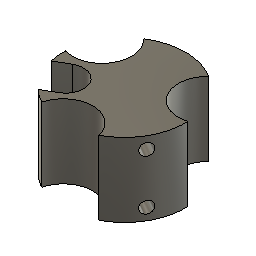
Holder UV v2 (Autodesk Fusion 360 design; units mm, degrees)
Autodesk Fusion 360 part; units mm, degrees
sketch "Sketch1" plane through (0, 0, 0) normal (0, 1, 0) x (1, 0, 0) in component "Holder UV"
  circle A0 centre (0, 0) radius 20.75
  line L0 (0, 0) -> (0, 20.75) construction
  line L1 (0, 0) -> (17.97, -10.375) construction
  line L2 (0, 0) -> (-17.97, -10.375) construction
  circle A1 centre (-12.6656, -7.3125) radius 6.125
  line L3 (-12.6656, -7.3125) -> (-15.7281, -2.0081)
  line L4 (-15.7281, -2.0081) -> (-20.2318, -4.6083)
  line L5 (-12.6656, -7.3125) -> (-9.6031, -12.6169)
  line L6 (-9.6031, -12.6169) -> (-14.1068, -15.2171)
  line L7 (17.97, 10.375) -> (0, -20.75)
  line L8 (0, -20.75) -> (-17.97, 10.375)
  line L9 (17.97, 10.375) -> (-17.97, 10.375)
  circle A2 centre (17.97, 10.375) radius 10
  circle A3 centre (-17.97, 10.375) radius 10
  circle A4 centre (0, -20.75) radius 10
  dimension "d1" = 41.5
  dimension "d4" = 120
  dimension "d5" = 120
  dimension "d6" = 12.25
  dimension "d7" = 6.125
  dimension "d8" = 20
  dimension "d10" = 360
  constraint coincident A0.centre L0.start
  constraint coincident A0 L0.end
  constraint vertical L0
  constraint coincident A0 L1.end
  constraint coincident A0 L2.end
  constraint coincident L2 A1.centre
  constraint coincident A1.centre L3.start
  constraint coincident A1 L3.end
  constraint perpendicular L2 L3
  constraint coincident A0 L4.end
  constraint tangent A1 L4
  constraint symmetric L2 A1.centre L3.start
  constraint symmetric L2 L3.end L5.end
  constraint symmetric L2 L4.end L6.end
  constraint coincident A0 L7.start
  constraint coincident A0 L7.end
  constraint perpendicular L1 L7
  constraint coincident A0 L8.end
  constraint perpendicular L2 L8
  constraint horizontal L9
  constraint coincident L7.start L9.start
  measures "d1" diameter of A0
  measures "d4" angle of L0 L1
  measures "d5" angle of L0 L2
  measures "d6" diameter of A1
  measures "d7" distance of L2.end A1.centre
  measures "d8" diameter of A2
extrude "Extrude1" add sketch "Sketch1" along normal blind 25 contours A0 L7 A2 A4 | A1 L7 L8 L9 A2 A3 A4 | A0 L9 A2 A3 | A0 A1 L6 L8 A4 | A0 A1 L4 L8 A3 in component "Holder UV"
ref_plane "WorkPlane1" through (17.97, 0, 10.375) normal (0.866025, 0, 0.5) x (0, 1, 0) in component "Holder UV"
sketch "Sketch2" plane through (17.97, 0, 10.375) normal (0.866025, 0, 0.5) x (0, 1, 0) in component "Holder UV"
  line L0 (0, -11.0305) -> (0, 11.0305)
  line L1 (0, -11.0305) -> (25, -11.0305)
  line L2 (25, -11.0305) -> (25, 11.0305)
  line L3 (25, 11.0305) -> (0, 11.0305)
  line L4 (0, 0) -> (25, 0) construction
  circle A0 centre (21, 0) radius 2
  circle A1 centre (4, 0) radius 2
  dimension "d11" = 4
  dimension "d12" = 4
  dimension "d13" = 4
  dimension "d14" = 4
  constraint coincident L4.start origin
  constraint midpoint L2 L4.end
  constraint coincident L4 A0.centre
  measures "d11" diameter of A0
  measures "d12" diameter of A1
  measures "d13" distance of A1.centre L4.start
  measures "d14" distance of L2 A0.centre
extrude "Extrude2" cut sketch "Sketch2" against normal blind 5 contours A0 | A1 in component "Holder UV"
ref_plane "WorkPlane2" through (0, 0, -20.75) normal (0, 0, -1) x (-1, 0, 0) in component "Holder UV"
sketch "Sketch3" plane through (0, 0, -20.75) normal (0, 0, -1) x (1, 0, 0) in component "Holder UV"
  line L0 (-11.0305, 0) -> (11.0305, 0)
  line L1 (-11.0305, 0) -> (-11.0305, -25)
  line L2 (-11.0305, -25) -> (11.0305, -25)
  line L3 (11.0305, -25) -> (11.0305, 0)
  line L4 (0, 0) -> (0, -25) construction
  circle A0 centre (0, -4) radius 2
  circle A1 centre (0, -21) radius 2
  line L5 (-20.75, 0) -> (20.75, 0)
  dimension "d17" = 4
  dimension "d18" = 4
  dimension "d19" = 4
  dimension "d20" = 4
  constraint coincident L4.start origin
  constraint midpoint L2 L4.end
  constraint coincident L4 A0.centre
  constraint coincident L4 A1.centre
  measures "d17" diameter of A0
  measures "d18" diameter of A1
  measures "d19" distance of A0.centre L5
  measures "d20" distance of L2 A1.centre
extrude "Extrude3" cut sketch "Sketch3" against normal blind 5 contours A0 | A1 in component "Holder UV"
component "Holder UV" placed x (1, 0, 0) y (0, 1, 0) z (0, 0, 1) at (0, 0, 0)
equation "d1 = 42 mm - 0.5 mm"
equation "d4 = ( 360 / 3 ) * 1 deg"
equation "d7 = ( 12.25 / 2 ) * 1 mm"
named bodies: "Holder UV"
